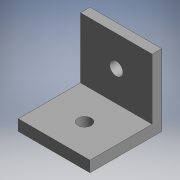
# Autodesk Inventor part: Part16
Saved by Autodesk Inventor 2016 (Build 200138000, 138)
## iProperties
Created: 2018-01-18
Part Number: Part16
Material: Generic
Document SubType Name: Modeling
Designer: student
Density: 1 g/cm^3
Appearance: Default
Author: student
Autodesk Inventor part; units mm, degrees
ref_plane "YZ Plane" through (0, 0, 0) normal (1, 0, 0) x (0, 1, 0)
ref_plane "XZ Plane" through (0, 0, 0) normal (0, 1, 0) x (-1, 0, 0)
ref_plane "XY Plane" through (0, 0, 0) normal (0, 0, 1) x (1, 0, 0)
sketch "Sketch1" plane through (0, 0, 0) normal (0, 1, 0) x (-1, 0, 0)
  line L0 (-13.4529, -30.7592) -> (5.5971, -30.7592)
  line L1 (5.5971, -30.7592) -> (5.5971, -49.8092)
  line L2 (5.5971, -49.8092) -> (-13.4529, -49.8092)
  line L3 (-13.4529, -49.8092) -> (-13.4529, -30.7592)
  line L4 (-13.4529, -30.7592) -> (5.5971, -49.8092) construction
  line L5 (5.5971, -30.7592) -> (-13.4529, -49.8092) construction
  line L6 (-3.9279, -30.7592) -> (-3.9279, -38.8592) construction
  circle A0 centre (-3.9279, -38.8592) radius 1.75
  point P0 (0, 0)
  point P1 (-3.9279, -40.2842)
  dimension "d0" = 19.05
  dimension "d1" = 19.05
  dimension "d8" = 8.1
  dimension "d9" = 3.5
  constraints: 14 end point, 3 midpoint, 2 parallel, 1 centre point, 1 coincident, 1 horizontal, 1 perpendicular, 1 vertical
  measures "d0" distance of L1.end L2.end
  measures "d1" distance of L0.end L1.end
  measures "d8" distance of L6.start L6.end
  measures "d9" diameter of A0
extrude "Extrusion1" add sketch "Sketch1" along normal blind 2.921
sketch "Sketch2" plane through (0, 2.921, 0) normal (0, 1, 0) x (1, 0, 0)
  line L0 (-5.5971, 49.8092) -> (13.4529, 49.8092)
  line L1 (13.4529, 49.8092) -> (13.4529, 47.2692)
  line L2 (13.4529, 47.2692) -> (-5.5971, 47.2692)
  line L3 (-5.5971, 47.2692) -> (-5.5971, 49.8092)
  point P0 (0, 0)
  dimension "d4" = 19.05
  dimension "d5" = 2.54
  constraints: 8 end point, 2 horizontal, 2 parallel, 1 perpendicular
  measures "d4" distance of L1.end L2.end
  measures "d5" distance of L0.end L1.end
extrude "Extrusion2" add sketch "Sketch2" along normal blind 16.129
sketch "Sketch3" plane through (13.4529, 0, -49.8092) normal (0, 0, -1) x (-1, 0, 0)
  line L0 (19.05, 0) -> (0, 0) construction
  line L1 (19.05, 0) -> (19.05, 19.05) construction
  line L2 (0, 19.05) -> (19.05, 19.05) construction
  line L3 (0, 0) -> (0, 19.05) construction
  line L4 (0, 19.05) -> (19.05, 19.05) construction
  line L5 (9.525, 19.05) -> (9.525, 10.95) construction
  circle A0 centre (9.525, 10.95) radius 1.75
  point P0 (13.4529, 0)
  dimension "d10" = 8.1
  dimension "d11" = 3.5
  constraints: 2 end point, 1 centre point, 1 coincident, 1 midpoint, 1 vertical
  measures "d10" distance of L5.start L5.end
  measures "d11" diameter of A0
extrude "Extrusion3" cut sketch "Sketch3" against normal blind 25.4
body "Solid1"
